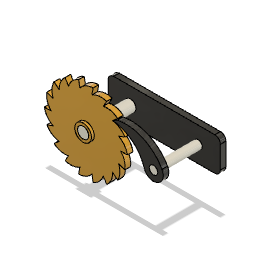
rachet_pawl (Autodesk Fusion 360 design; units mm, degrees)
Autodesk Fusion 360 part; units mm, degrees
note: some values were not read from the file. Set by a fixed rule: which sketch regions a step uses.
sketch "Sketch1" plane through (0, 0, 0) normal (0, 0, 1) x (1, 0, 0)
  circle A0 centre (-37.8029, 150.2074) radius 62.5
  circle A1 centre (-37.8029, 150.2074) radius 75
  line L0 (-37.8029, 150.2074) -> (-37.8029, 225.2074)
  line L1 (-37.8029, 150.2074) -> (-48.6559, 211.7579)
  line L2 (-37.8029, 150.2074) -> (24.6971, 150.2074) construction
  line L3 (-37.8029, 150.2074) -> (-24.8555, 223.6361)
  line L4 (-37.8029, 150.2074) -> (37.1971, 150.2074) construction
  arc A2 (-24.8555, 223.6361) -> (-48.6559, 211.7579) centre (-24.7476, 193.6363) ccw
  circle A3 centre (-37.8029, 150.2074) radius 15
  circle A4 centre (-37.8029, 150.2074) radius 10
  dimension "d1" = 125
  dimension "d2" = 12.5
  dimension "d3" = 100
  dimension "d4" = 62.5
  dimension "d5" = 80
  dimension "d6" = 30
  dimension "d8" = 30
  dimension "d9" = 20
  constraint coincident A0.centre A1.centre
  constraint coincident A1 L0.end
  constraint vertical L0
  constraint horizontal L2
  constraint horizontal L4
  measures "d1" diameter of A0
  measures "d3" angle of L1 L2
  measures "d4" distance of A0.centre L1.end
  measures "d5" angle of L3 L4
  measures "d6" radius of A2
  measures "d8" diameter of A3
  measures "d9" diameter of A4
extrude "Extrude1" add sketch "Sketch1" along normal mid plane 10 contours A0 L0 A2 | A0 L0 L1 A3 | A0 L0 L3 A2 | A0 L0 L3 A3 makes body 1
pattern_circular "C-Pattern1" count 18 over 360 about axis through (-37.8029, 150.2074, 5) along (0, 0, -1) of bodies 1 makes body 2 at (-19.2583, 196.5784, 5) makes body 3 at (-4.5169, 187.4393, 5) makes body 4 at (6.2097, 173.8094, -5) makes body 5 at (11.6278, 157.3328, 5) makes body 6 at (11.0838, 139.9968, 5) makes body 7 at (4.6434, 123.8923, 5) makes body 8 at (-6.9168, 110.9619, 5) makes body 9 at (-22.2022, 102.765, 5) makes body 10 at (-39.3693, 100.2903, 5) makes body 11 at (-56.3475, 103.8364, 5) makes body 12 at (-71.0889, 112.9756, -5) makes body 13 at (-81.8156, 126.6054, 5) makes body 14 at (-87.2337, 143.082, 5) makes body 15 at (-86.6897, 160.418, 5) makes body 16 at (-80.2492, 176.5225, 5) makes body 17 at (-68.6891, 189.453, 5) makes body 18 at (-53.4036, 197.6499, 5)
extrude "Extrude2" add sketch "Sketch1" along normal mid plane 20 contours L0 L1 A3 A4 | L1 L3 A3 A4 | L0 L3 A3 A4 bodies 1 2 3 4 5 6 7 8 9 10 11 12 13 14 15 16 17 18
copy_body "Body->Comp1" bodies 1 removing the originals makes body 19 in component "Component"
sketch "Sketch2" plane through (0, 0, 0) normal (0, 0, 1) x (1, 0, 0)
  circle A0 centre (-37.8029, 150.2074) radius 10
  circle A1 centre (-37.8029, 150.2074) radius 15
  line L0 (-48.6559, 211.7579) -> (-50.7504, 223.6361)
  arc A2 (-50.7504, 223.6361) -> (-69.0529, 204.334) centre (-40.3885, 195.4824) ccw
  line L1 (-69.0529, 204.334) -> (-75.0836, 214.7795)
  arc A3 (-75.0836, 214.7795) -> (-85.6807, 190.3817) centre (-55.7175, 191.8677) ccw
  line L2 (-85.6807, 190.3817) -> (-94.9203, 198.1346)
  arc A4 (-94.9203, 198.1346) -> (-96.5337, 171.5837) centre (-68.8858, 183.2281) ccw
  line L3 (-96.5337, 171.5837) -> (-107.8678, 175.7089)
  arc A5 (-107.8678, 175.7089) -> (-100.3029, 150.2074) centre (-78.305, 170.6057) ccw
  line L4 (-100.3029, 150.2074) -> (-112.3644, 150.2074)
  arc A6 (-112.3644, 150.2074) -> (-96.5337, 128.8312) centre (-82.839, 155.523) ccw
  line L5 (-96.5337, 128.8312) -> (-107.8678, 124.7059)
  arc A7 (-107.8678, 124.7059) -> (-85.6807, 110.0332) centre (-81.9411, 139.7992) ccw
  line L6 (-85.6807, 110.0332) -> (-94.9203, 102.2803)
  arc A8 (-94.9203, 102.2803) -> (-69.0529, 96.0808) centre (-75.7194, 125.3308) ccw
  line L7 (-69.0529, 96.0808) -> (-75.0836, 85.6353)
  arc A9 (-75.0836, 85.6353) -> (-48.6559, 88.6569) centre (-64.9244, 113.8628) ccw
  line L8 (-48.6559, 88.6569) -> (-50.7504, 76.7787)
  arc A10 (-50.7504, 76.7787) -> (-26.9499, 88.6569) centre (-50.8582, 106.7785) ccw
  line L9 (-26.9499, 88.6569) -> (-24.8555, 76.7787)
  arc A11 (-24.8555, 76.7787) -> (-6.5529, 96.0808) centre (-35.2173, 104.9325) ccw
  line L10 (-6.5529, 96.0808) -> (-0.5222, 85.6353)
  arc A12 (-0.5222, 85.6353) -> (10.0749, 110.0332) centre (-19.8883, 108.5472) ccw
  line L11 (10.0749, 110.0332) -> (19.3145, 102.2803)
  arc A13 (19.3145, 102.2803) -> (20.9279, 128.8312) centre (-6.7201, 117.1868) ccw
  line L12 (20.9279, 128.8312) -> (32.2619, 124.7059)
  arc A14 (32.2619, 124.7059) -> (24.6971, 150.2074) centre (2.6991, 129.8091) ccw
  line L13 (24.6971, 150.2074) -> (36.7585, 150.2074)
  arc A15 (36.7585, 150.2074) -> (20.9279, 171.5837) centre (7.2332, 144.8918) ccw
  line L14 (20.9279, 171.5837) -> (32.2619, 175.7089)
  arc A16 (32.2619, 175.7089) -> (10.0749, 190.3817) centre (6.3352, 160.6156) ccw
  line L15 (10.0749, 190.3817) -> (19.3145, 198.1346)
  arc A17 (19.3145, 198.1346) -> (-6.5529, 204.334) centre (0.1136, 175.0841) ccw
  line L16 (-6.5529, 204.334) -> (-0.5222, 214.7795)
  arc A18 (-0.5222, 214.7795) -> (-26.9499, 211.7579) centre (-10.6814, 186.552) ccw
  line L17 (-26.9499, 211.7579) -> (-24.8555, 223.6361)
  arc A19 (-24.8555, 223.6361) -> (-48.6559, 211.7579) centre (-24.7476, 193.6363) ccw
  circle A20 centre (83.6452, 150.2074) radius 17.5
  arc A21 (66.9426, 144.985) -> (10.0749, 190.3817) centre (4.9044, 125.5876) ccw
  circle A22 centre (83.6452, 150.2074) radius 7.5
  line L18 (10.0749, 190.3817) -> (18.7351, 195.3817)
  line L19 (10.0749, 190.3817) -> (20.0749, 190.3817) construction
  arc A23 (98.8728, 158.8313) -> (18.7351, 195.3817) centre (33.6117, 121.8719) ccw
  dimension "d16" = 35
  dimension "d17" = 65
  dimension "d19" = 15
  dimension "d44" = 30
  dimension "d45" = 10
  dimension "d46" = 75
  constraint coincident A20 A21.start
  constraint coincident A16.end L15.start
  constraint tangent A20 A21
  constraint concentric A20 A22
  constraint horizontal L19
  constraint coincident A20 A23.start
  constraint tangent A20 A23
  measures "d16" diameter of A20
  measures "d17" radius of A21
  measures "d19" diameter of A22
  measures "d44" angle of L18 L19
  measures "d45" distance of A16.end L18.end
  measures "d46" radius of A23
extrude "Extrude1'" add sketch "Sketch2" along normal mid plane 10 separate body contours A20 A21 L18 A23 | A20 makes body 20 in component "Component'"
sketch "Sketch3" plane through (0, 0, 5) normal (0, 0, 1) x (1, 0, 0)
  circle A0 centre (83.6452, 150.2074) radius 7.5
  line L0 (-67.8029, 180.2074) -> (113.6452, 180.2074)
  line L1 (123.6452, 170.2074) -> (123.6452, 130.2074)
  line L2 (113.6452, 120.2074) -> (-67.8029, 120.2074)
  line L3 (-77.8029, 130.2074) -> (-77.8029, 170.2074)
  circle A1 centre (-37.8029, 150.2074) radius 10
  circle A2 centre (83.6452, 150.2074) radius 7.5
  arc A3 (-67.8029, 180.2074) -> (-77.8029, 170.2074) centre (-67.8029, 170.2074) ccw
  arc A4 (-77.8029, 130.2074) -> (-67.8029, 120.2074) centre (-67.8029, 130.2074) ccw
  arc A5 (123.6452, 170.2074) -> (113.6452, 180.2074) centre (113.6452, 170.2074) ccw
  arc A6 (113.6452, 120.2074) -> (123.6452, 130.2074) centre (113.6452, 130.2074) ccw
  arc A7 (66.9426, 144.985) -> (98.8728, 158.8313) centre (83.6452, 150.2074) ccw
  arc A8 (98.8728, 158.8313) -> (18.7351, 195.3817) centre (33.6117, 121.8719) ccw
  line L4 (18.7351, 195.3817) -> (10.0749, 190.3817)
  arc A9 (66.9426, 144.985) -> (10.0749, 190.3817) centre (4.9044, 125.5876) ccw
  dimension "d22" = 40
  dimension "d23" = 30
  dimension "d24" = 30
  dimension "d25" = 40
  dimension "d26" = 10
  constraint horizontal L0
  constraint vertical L1
  constraint horizontal L2
  constraint vertical L3
  constraint tangent L0 A3
  constraint tangent L3 A3
  constraint tangent L2 A4
  constraint tangent L3 A4
  constraint equal A3 A4
  constraint tangent L0 A5
  constraint tangent L1 A5
  constraint equal A3 A5
  constraint tangent L1 A6
  constraint tangent L2 A6
  constraint equal A3 A6
  measures "d22" distance of L3 A1.centre
  measures "d23" distance of L0 A1.centre
  measures "d24" distance of L2 A1.centre
  measures "d25" distance of L1 A0.centre
  measures "d26" radius of A3
extrude "Extrude3" add sketch "Sketch3" against normal blind 10 from surface at -80 separate body contours L0 L1 L2 L3 A3 A4 A5 A6 A7 A8 A9 | L0 A7 A8 A9 makes body 21
copy_body "Body->Comp2" bodies 21 removing the originals makes body 22 in component "Component''"
extrude "Extrude1''" add sketch "Sketch3" against normal blind 90 separate body contours A0 A2 | A1 makes body 23 at (90.9133, 152.0581, -55) makes body 24 at (-27.8154, 149.709, -55) in component "Component'''"
move_face "OffsetFaces1" offset 5 1 faces at (-40.9509, 149.7217, 5) on bodies 24 in component "Component'''"
copy_body "Body->Comp1'" bodies 23 removing the originals makes body 25 in component "Component''''"
copy_body "Body->Comp2'" bodies 24 removing the originals makes body 26 in component "Component'''''"
component "Component" placed x (1, 0, 0) y (0, 1, 0) z (0, 0, 1) at (0, 0, 0)
component "Component'" placed x (1, 0, 0) y (0, 1, 0) z (0, 0, 1) at (0, 0, 0)
component "Component''" placed x (1, 0, 0) y (0, 1, 0) z (0, 0, 1) at (0, 0, 0)
component "Component'''''" placed x (1, 0, 0) y (0, 1, 0) z (0, 0, 1) at (0, 0, 0) in component "Component''"
component "Component''''" placed x (1, 0, 0) y (0, 1, 0) z (0, 0, 1) at (0, 0, 0) in component "Component''"
